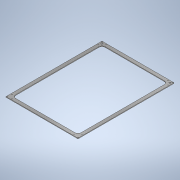
# Autodesk Inventor part: top_plate
Saved by Autodesk Inventor 2021 (Build 250183000, 183)
## iProperties
Created: 2023-01-13
Part Number: top_plate
Material: Типовые
Document SubType Name: Modeling
Designer: ignat
Density: 1 g/cm^3
Appearance: По умолчанию
Author: ignat
Autodesk Inventor part; units mm, degrees
ref_plane "YZ Plane" through (0, 0, 0) normal (1, 0, 0) x (0, 1, 0)
ref_plane "XZ Plane" through (0, 0, 0) normal (0, 1, 0) x (-1, 0, 0)
ref_plane "XY Plane" through (0, 0, 0) normal (0, 0, 1) x (1, 0, 0)
sketch "Эскиз1" plane through (0, 0, 0) normal (0, 1, 0) x (-1, 0, 0)
  line L0 (-260, 375) -> (190, 375)
  line L1 (190, 375) -> (190, -225)
  line L2 (190, -225) -> (-260, -225)
  line L3 (-260, -225) -> (-260, 375)
  line L4 (-260, 375) -> (190, -225) construction
  line L5 (190, 375) -> (-260, -225) construction
  circle A0 centre (-228.75, 368.75) radius 1.75
  circle A1 centre (-253.75, 343.75) radius 1.75
  circle A2 centre (-256, 371) radius 1.75
  circle A3 centre (186, 371) radius 1.75
  circle A4 centre (183.75, 343.75) radius 1.75
  circle A5 centre (158.75, 368.75) radius 1.75
  circle A6 centre (183.75, -193.75) radius 1.75
  circle A7 centre (186, -221) radius 1.75
  circle A8 centre (158.75, -218.75) radius 1.75
  circle A9 centre (-253.75, -193.75) radius 1.75
  circle A10 centre (-256, -221) radius 1.75
  circle A11 centre (-228.75, -218.75) radius 1.75
  line L6 (170, -205) -> (170, 355)
  line L7 (170, 355) -> (-240, 355)
  line L8 (-240, 355) -> (-240, -205)
  line L9 (-240, -205) -> (170, -205)
  point P0 (0, 0)
  dimension "d0" = 450
  dimension "d1" = 600
  dimension "d11" = 20
  dimension "d21" = 27.25
  dimension "d22" = 2.25
  dimension "d23" = 27.25
  dimension "d24" = 2.25
  dimension "d25" = 4
  dimension "d26" = 4
  dimension "d27" = 27.25
  dimension "d28" = 4
  dimension "d29" = 4
  dimension "d30" = 27.25
  dimension "d31" = 2.25
  dimension "d32" = 2.25
  dimension "d34" = 27.25
  dimension "d35" = 27.25
  dimension "d36" = 2.25
  dimension "d37" = 2.25
  dimension "d38" = 4
  dimension "d39" = 4
  dimension "d40" = 27.25
  dimension "d41" = 27.25
  dimension "d42" = 2.25
  dimension "d43" = 2.25
  dimension "d44" = 4
  dimension "d45" = 4
  constraints: 20 end point, 12 centre point, 4 parallel, 2 perpendicular, 1 horizontal, 3 other
  measures "d0" distance of L2.start L2.end
  measures "d1" distance of L1.start L2.start
  measures "d11" distance between parallel lines of L1 L6
  measures "d21" vertical distance of A3.centre A4.centre
  measures "d22" horizontal distance of A3.centre A4.centre
  measures "d23" horizontal distance of A5.centre A3.centre
  measures "d24" vertical distance of A5.centre A3.centre
  measures "d25" distance from line of L0 A3.centre
  measures "d26" distance from line of L1 A3.centre
  measures "d27" horizontal distance of A2.centre A0.centre
  measures "d28" distance from line of L3 A2.centre
  measures "d29" distance from line of L0 A2.centre
  measures "d30" vertical distance of A2.centre A1.centre
  measures "d31" horizontal distance of A2.centre A1.centre
  measures "d32" vertical distance of A0.centre A2.centre
  measures "d34" vertical distance of A7.centre A6.centre
  measures "d35" horizontal distance of A8.centre A7.centre
  measures "d36" vertical distance of A7.centre A8.centre
  measures "d37" horizontal distance of A6.centre A7.centre
  measures "d38" distance from line of L1 A7.centre
  measures "d39" distance from line of A7.centre L2
  measures "d40" vertical distance of A10.centre A9.centre
  measures "d41" horizontal distance of A11.centre A10.centre
  measures "d42" horizontal distance of A9.centre A10.centre
  measures "d43" vertical distance of A11.centre A10.centre
  measures "d44" distance from line of L2 A10.centre
  measures "d45" distance from line of A10.centre L3
extrude "Выдавливание1" add sketch "Эскиз1" along normal blind 4
fillet "Сопряжение1" radius 20 4 edges at (240, 2, -205) (-170, 2, -205) (-170, 2, 355) (240, 2, 355)
sketch "Эскиз2" plane through (0, 4, 0) normal (0, 1, 0) x (1, 0, 0)
  circle A0 centre (-177.5, 212.5) radius 7 projected
  circle A1 centre (247.5, 212.5) radius 7 projected
  circle A2 centre (247.5, -362.5) radius 7 projected
  circle A3 centre (-177.5, -362.5) radius 7 projected
  circle A4 centre (-177.5, -362.5) radius 5
  circle A5 centre (247.5, -362.5) radius 5
  circle A6 centre (247.5, 212.5) radius 5
  circle A7 centre (-177.5, 212.5) radius 5
  line L0 (260, 225) -> (-190, 225) projected
  point P0 (0, 0)
  dimension "d15" = 10
  dimension "d16" = 10
  dimension "d17" = 10
  dimension "d18" = 10
  dimension "d33" = 12.5
  constraints: 4 centre point, 4 coincident
  measures "d15" diameter of A4
  measures "d16" diameter of A5
  measures "d17" diameter of A6
  measures "d18" diameter of A7
  measures "d33" distance from line of L0 A0.centre
extrude "Выдавливание2" cut sketch "Эскиз2" against normal through all contours A4 | A5 | A6 | A7
